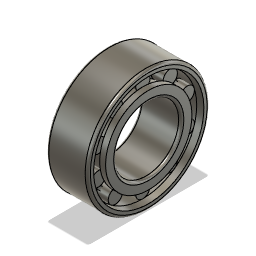
Bearing_GOST_7634-75_282000 (Autodesk Fusion 360 design; units mm, degrees)
Autodesk Fusion 360 part; units mm, degrees
note: some values were not read from the file. Chosen so that the rebuilt part matches the saved one: which bodies a step acts on.
sketch "Sketch1" plane through (0, 0, 0) normal (0, 0, 1) x (1, 0, 0)
  line L0 (-85, 0) -> (85, 0)
  line L1 (-8, 12.5) -> (8, 12.5)
  line L2 (8, 12.5) -> (8, 16.625)
  line L3 (-8, 12.5) -> (-8, 16.625)
  line L4 (-8, 16.625) -> (-5.7143, 16.625)
  line L5 (-5.7143, 16.625) -> (-5.7143, 15.25)
  line L6 (-5.7143, 15.25) -> (-1.1429, 15.25)
  line L7 (-1.1429, 15.25) -> (-1.1429, 16.625)
  line L8 (-1.1429, 16.625) -> (1.1429, 16.625)
  line L9 (1.1429, 16.625) -> (1.1429, 15.25)
  line L10 (1.1429, 15.25) -> (5.7143, 15.25)
  line L11 (5.7143, 15.25) -> (5.7143, 16.625)
  line L12 (5.7143, 16.625) -> (8, 16.625)
  line L13 (-8, 21.2358) -> (-5.7143, 20.75)
  line L14 (-5.7143, 20.75) -> (5.7143, 20.75)
  line L15 (5.7143, 20.75) -> (8, 21.2358)
  line L16 (8, 21.2358) -> (8, 23.5)
  line L17 (8, 23.5) -> (-8, 23.5)
  line L18 (-8, 23.5) -> (-8, 21.2358)
  line L19 (5.7143, 20.75) -> (5.7143, 16.625)
  line L20 (1.1429, 16.625) -> (1.1429, 20.75)
  line L21 (-1.1429, 16.625) -> (-1.1429, 20.75)
  line L22 (-5.7143, 16.625) -> (-5.7143, 20.75)
  line L23 (-3.4286, 20.75) -> (-3.4286, 15.25) construction
  line L24 (-5.7143, 18) -> (-1.1429, 18)
  line L25 (3.4286, 20.75) -> (3.4286, 15.25) construction
  line L26 (1.1429, 18) -> (5.7143, 18)
  line L27 (-2.2857, 18.6875) -> (2.2857, 18.6875)
  line L28 (2.2857, 18.6875) -> (2.2857, 17.3125)
  line L29 (2.2857, 17.3125) -> (-2.2857, 17.3125)
  line L30 (-2.2857, 17.3125) -> (-2.2857, 18.6875)
  point P0 (0, 16.625)
  point P1 (0, 23.5)
  point P2 (-3.4286, 18)
  point P3 (3.4286, 18)
  point P4 (-2.2857, 18)
  point P5 (2.2857, 18)
  point P6 (0, 18.6875)
  dimension "d1" = 12
  dimension "d2" = 12
  dimension "d3" = 47
  dimension "d4" = 25
  dimension "d5" = 2.2857
  dimension "d6" = 4.5714
  dimension "d7" = 16
  dimension "d8" = 5.5
  dimension "d10" = 5.5
  dimension "d11" = 2.75
  dimension "d19" = 4.5714
  dimension "d20" = 1.375
  constraint horizontal L0
  constraint midpoint L0 origin
  constraint vertical L2
  constraint vertical L3
  constraint perpendicular L3 L4
  constraint perpendicular L4 L5
  constraint perpendicular L5 L6
  constraint perpendicular L4 L7
  constraint perpendicular L7 L8
  constraint perpendicular L8 L9
  constraint perpendicular L9 L10
  constraint perpendicular L8 L11
  constraint perpendicular L2 L12
  constraint horizontal L14
  constraint perpendicular L14 L16
  constraint perpendicular L16 L17
  constraint perpendicular L17 L18
  constraint vertical L2.end L15.end
  constraint vertical L3.end L13.start
  constraint midpoint L8 P0
  constraint midpoint L17 P1
  constraint vertical P0 P1
  constraint vertical origin P0
  constraint horizontal L4.end L7.end
  constraint horizontal L8.end L11.end
  constraint equal L6 L10
  constraint vertical L4.end L13.end
  constraint vertical L11.end L14.end
  constraint coincident L14 L20.end
  constraint perpendicular L14 L20
  constraint coincident L14 L21.end
  constraint perpendicular L14 L21
  constraint perpendicular L14 L22
  constraint coincident L14 L23.start
  constraint midpoint L6 L23.end
  constraint perpendicular L6 L23
  constraint midpoint L23 P2
  constraint coincident L22 L24.start
  constraint coincident L21 L24.end
  constraint perpendicular L21 L24
  constraint coincident P2 L24
  constraint coincident L14 L25.start
  constraint midpoint L10 L25.end
  constraint perpendicular L10 L25
  constraint coincident L20 L26.start
  constraint coincident L19 L26.end
  constraint perpendicular L19 L26
  constraint midpoint L25 P3
  constraint coincident L26 P3
  constraint horizontal L6.end L9.end
  constraint horizontal L27
  constraint vertical L28
  constraint horizontal L29
  constraint vertical L30
  constraint midpoint L30 P4
  constraint midpoint L28 P5
  constraint coincident L24 P4
  constraint midpoint L27 P6
  constraint vertical P0 P6
  constraint perpendicular L1 L2
  measures "d1" angle of L13 L14
  measures "d2" angle of L14 L15
  measures "d5" distance of L7 L9
  measures "d6" distance of L5 L7
  measures "d7" distance of L16 L18
  measures "d8" distance of L6 L14
  measures "d10" vertical distance of L1.start L24.start
  measures "d19" distance of L28.end L29.end
  measures "d20" distance of L27.end L28.end
revolve "Revolve1" add sketch "Sketch1" angle 360 about axis through (-85, 0, 0) along (1, 0, 0) contours L1 L2 L3 L4 L5 L6 L7 L8 L9 L10 L11 L12 | L13 L14 L15 L16 L17 L18 makes body 1 at (2.6667, 12.4845, -0.6231) makes body 2 at (2.6667, 23.4708, -1.1714)
revolve "Revolve2" add sketch "Sketch1" angle 360 about axis through (-5.7143, 18, 0) along (1, 0, 0) separate body contours L5 L6 L7 L21 L22 L24 L29 L30 | L9 L10 L11 L19 L20 L26 L28 L29 | L21 L24 L29 L30 | L20 L26 L28 L29 makes body 3 at (-4.1905, 15.2534, 0.1371) makes body 4 at (2.6667, 15.2534, 0.1371)
fillet "Fillet1" radius 1 4 edges at (8, -4.5202, 11.6541) (-8, -4.5202, 11.6541) (-8, -8.498, 21.9097) (8, -8.498, 21.9097) on bodies 1 2
pattern_circular "C-Pattern1" count 10 over 360 about axis through (-85, 0, 0) along (1, 0, 0) of bodies 3 4 makes body 5 at (-4.1905, 12.2597, 9.0766) makes body 6 at (-4.1905, 4.5832, 14.5492) makes body 7 at (-2.6667, -4.9771, 14.432) makes body 8 at (-4.1905, -12.4208, 8.8548) makes body 9 at (-4.1905, -15.2534, -0.1371) makes body 10 at (-4.1905, -12.2597, -9.0766) makes body 11 at (-4.1905, -4.5832, -14.5492) makes body 12 at (2.6667, 12.2597, 9.0766) makes body 13 at (2.6667, 4.5832, 14.5492) makes body 14 at (2.6667, -4.8439, 14.4645) makes body 15 at (2.6667, -12.4208, 8.8548) makes body 16 at (2.6667, -15.2534, -0.1371) makes body 17 at (2.6667, -12.2597, -9.0766) makes body 18 at (2.6667, -4.5832, -14.5492) makes body 19 at (-4.1905, 4.8439, -14.4645) makes body 20 at (-4.1905, 12.4208, -8.8548) makes body 21 at (2.6667, 4.8439, -14.4645) makes body 22 at (2.6667, 12.4208, -8.8548)
revolve "Revolve3" add sketch "Sketch1" angle 360 about axis through (-85, 0, 0) along (1, 0, 0) separate body contours L21 L24 L27 L30 | L21 L24 L29 L30 | L20 L26 L28 L29 | L20 L26 L27 L28 | L20 L21 L27 L29 makes body 23
